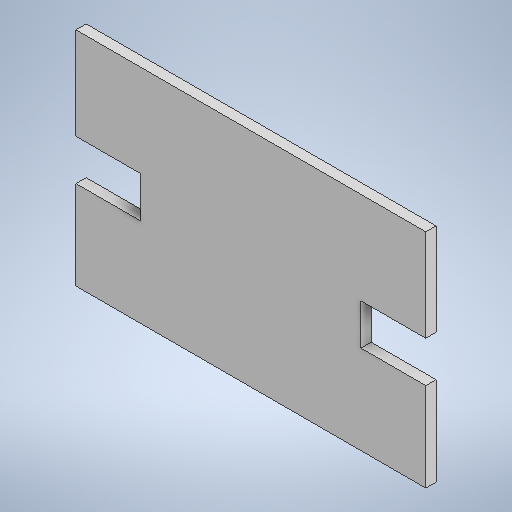
# Autodesk Inventor part: carcasa_piezaFrontal
Saved by Autodesk Inventor 2025.3 (Build 293356030, 356C)
## iProperties
Created: 2025-09-08
Part Number: carcasa_piezaFrontal
Material: Generic
Document SubType Name: Modeling
Designer: brene
Density: 1 g/cm^3
Appearance: Default
Author: brene
Autodesk Inventor part; units mm, degrees
ref_plane "YZ Plane" through (0, 0, 0) normal (1, 0, 0) x (0, 1, 0)
ref_plane "XZ Plane" through (0, 0, 0) normal (0, 1, 0) x (-1, 0, 0)
ref_plane "XY Plane" through (0, 0, 0) normal (0, 0, 1) x (1, 0, 0)
sketch "Sketch1" plane through (0, 0, 0) normal (0, 0, 1) x (1, 0, 0)
  line L0 (0, 0) -> (102.47, 0)
  line L1 (102.47, 0) -> (102.47, 65)
  line L2 (102.47, 65) -> (0, 65)
  line L3 (0, 65) -> (0, 0)
  dimension "d0" = 102.47
  dimension "d1" = 65
  constraints: 8 end point, 2 perpendicular, 1 horizontal, 1 parallel
  measures "d0" distance of L0.start L0.end
  measures "d1" distance of L0.end L1.end
extrude "Extrusion1" add sketch "Sketch1" along normal blind 3
sketch "Sketch2" plane through (0, 0, 3) normal (0, 0, 1) x (1, 0, 0)
  line L0 (0, 0) -> (102.47, 0) projected
  line L1 (51.235, 0) -> (51.235, 65)
  line L2 (102.47, 0) -> (102.47, 26)
  line L3 (102.47, 0) -> (102.47, 65) projected
  line L4 (102.47, 26) -> (83.47, 26)
  line L5 (83.47, 26) -> (83.47, 38)
  line L6 (83.47, 38) -> (102.47, 38)
  line L7 (0, 0) -> (0, 26)
  line L8 (0, 26) -> (19, 26)
  line L9 (19, 26) -> (19, 38)
  line L10 (19, 38) -> (0, 38)
  line L11 (0, 26) -> (0, 38)
  line L12 (0, 65) -> (0, 0) projected
  dimension "d8" = 26
  dimension "d9" = 19
  dimension "d10" = 12
  dimension "d11" = 19
  constraints: 20 end point, 4 symmetric about line, 2 perpendicular, 2 point on line, 1 collinear, 1 midpoint, 1 vertical
  measures "d8" distance of L0.end L2.end
  measures "d9" distance of L2.end L4.end
  measures "d10" distance of L4.end L5.end
  measures "d11" distance of L5.end L6.end
extrude "Extrusion2" cut sketch "Sketch2" against normal blind 50.975
body "Solid1"
